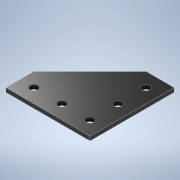
# Autodesk Inventor part: RightAngle_SideBracket
Saved by Autodesk Inventor 2021 (Build 250183000, 183)
## iProperties
Created: 2021-10-08
Part Number: RightAngle_SideBracket
Material: Generic
Document SubType Name: Modeling
Designer: Jorian Brusind
Density: 1 g/cm^3
Appearance: Glossy - Black
Author: Jorian Brusind
Autodesk Inventor part; units mm, degrees
ref_plane "YZ Plane" through (0, 0, 0) normal (1, 0, 0) x (0, 1, 0)
ref_plane "XZ Plane" through (0, 0, 0) normal (0, 1, 0) x (-1, 0, 0)
ref_plane "XY Plane" through (0, 0, 0) normal (0, 0, 1) x (1, 0, 0)
sketch "Sketch1" plane through (0, 0, 0) normal (0, 1, 0) x (-1, 0, 0)
  line L0 (0, 0) -> (60, 0)
  line L1 (0, 0) -> (60, 0) construction
  line L2 (0, 0) -> (0, -60)
  line L3 (0, -60) -> (20, -60)
  line L4 (60, 0) -> (60, -20)
  line L5 (60, -20) -> (20, -60)
  circle A0 centre (10, -10) radius 2.75
  circle A1 centre (30, -10) radius 2.75
  circle A2 centre (50, -10) radius 2.75
  circle A3 centre (10, -30) radius 2.75
  circle A4 centre (10, -50) radius 2.75
  dimension "d0" = 60
  dimension "d1" = 0
  dimension "d2" = 60
  dimension "d3" = 20
  dimension "d4" = 20
  dimension "d5" = 5.5
  dimension "d6" = 10
  dimension "d7" = 10
  dimension "d10" = 20
  dimension "d17" = 20
  constraints: 12 end point, 5 centre point, 3 horizontal, 2 perpendicular, 2 vertical, 1 collinear, 8 other
  measures "d0" distance of L0.start L0.end
  measures "d1" distance between parallel lines of L0 L1
  measures "d2" distance of L0.start L2.end
  measures "d3" distance of L2.end L3.end
  measures "d4" distance of L1.end L4.end
  measures "d5" diameter of A0
  measures "d6" distance from line of L2 A0.centre
  measures "d7" distance from line of L0 A0.centre
  measures "d10" distance of A0.centre A1.centre
  measures "d17" distance of A0.centre A3.centre
extrude "Extrusion1" add sketch "Sketch1" along normal blind 3
body "Solid1"
